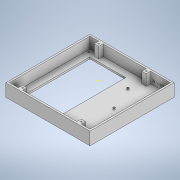
# Autodesk Inventor part: Backbox
Saved by Autodesk Inventor 2021 (Build 250183000, 183)
## iProperties
Created: 2022-08-07
Part Number: Backbox
Material: Generic
Document SubType Name: Modeling
Designer: Solom
Density: 1 g/cm^3
Appearance: Default
Author: Solom
Autodesk Inventor part; units mm, degrees
ref_plane "YZ Plane" through (0, 0, 0) normal (1, 0, 0) x (0, 1, 0)
ref_plane "XZ Plane" through (0, 0, 0) normal (0, 1, 0) x (-1, 0, 0)
ref_plane "XY Plane" through (0, 0, 0) normal (0, 0, 1) x (1, 0, 0)
sketch "Sketch1" plane through (0, 0, 0) normal (0, 1, 0) x (-1, 0, 0)
  line L0 (101.9092, 109.3301) -> (-90.0908, 109.3301)
  line L1 (-90.0908, 109.3301) -> (-90.0908, -82.6699)
  line L2 (-90.0908, -82.6699) -> (101.9092, -82.6699)
  line L3 (101.9092, -82.6699) -> (101.9092, 109.3301)
  line L4 (81.9092, 89.3301) -> (-70.0908, 89.3301)
  line L5 (-70.0908, 89.3301) -> (-70.0908, -62.6699)
  line L6 (-70.0908, -62.6699) -> (81.9092, -62.6699)
  line L7 (81.9092, -62.6699) -> (81.9092, 89.3301)
  point P0 (0, 0)
  dimension "d0" = 192
  dimension "d1" = 192
  dimension "d2" = 152
  dimension "d3" = 152
  dimension "d4" = 20
  dimension "d5" = 20
  constraints: 16 end point, 4 parallel, 2 horizontal, 2 perpendicular
  measures "d0" distance of L2.end L1.end
  measures "d1" distance of L1.end L0.end
  measures "d2" distance of L6.end L5.end
  measures "d3" distance of L5.end L4.end
  measures "d4" distance between parallel lines of L7 L3
  measures "d5" distance between parallel lines of L2 L6
extrude "Extrusion1" add sketch "Sketch1" along normal blind 4
sketch "Sketch2" plane through (0, 4, 0) normal (0, 1, 0) x (1, 0, 0)
  circle A0 centre (-92.4092, -96.8301) radius 1.5
  line L0 (-101.9092, -109.3301) -> (90.0908, -109.3301) projected
  line L1 (-101.9092, 82.6699) -> (-101.9092, -109.3301) projected
  circle A1 centre (-92.4092, 70.1699) radius 1.5
  line L2 (90.0908, 82.6699) -> (-101.9092, 82.6699) projected
  circle A2 centre (80.5908, 70.1699) radius 1.5
  line L3 (90.0908, -109.3301) -> (90.0908, 82.6699) projected
  circle A3 centre (80.5908, -96.8301) radius 1.5
  line L4 (-96.9092, 77.6699) -> (85.0908, 77.6699)
  line L5 (85.0908, 77.6699) -> (85.0908, -104.3301)
  line L6 (85.0908, -104.3301) -> (-96.9092, -104.3301)
  line L7 (-96.9092, -104.3301) -> (-96.9092, 77.6699)
  circle A4 centre (-84.4092, -101.8301) radius 1.25
  circle A5 centre (72.5908, 75.1699) radius 1.25
  point P0 (0, 0)
  dimension "d8" = 3
  dimension "d9" = 12.5
  dimension "d10" = 9.5
  dimension "d11" = 3
  dimension "d12" = 9.5
  dimension "d13" = 12.5
  dimension "d14" = 3
  dimension "d15" = 12.5
  dimension "d16" = 9.5
  dimension "d17" = 3
  dimension "d18" = 5
  dimension "d19" = 5
  dimension "d20" = 5
  dimension "d21" = 5
  dimension "d22" = 2.5
  dimension "d25" = 17.5
  dimension "d26" = 7.5
  dimension "d27" = 2.5
  dimension "d28" = 17.5
  dimension "d29" = 7.5
  constraints: 8 end point, 6 centre point, 2 parallel, 1 horizontal, 1 perpendicular
  measures "d8" diameter of A0
  measures "d9" distance from line of L0 A0.centre
  measures "d10" distance from line of L1 A0.centre
  measures "d11" diameter of A1
  measures "d12" distance from line of A1.centre L1
  measures "d13" distance from line of L2 A1.centre
  measures "d14" diameter of A2
  measures "d15" distance from line of L2 A2.centre
  measures "d16" distance from line of L3 A2.centre
  measures "d17" diameter of A3
  measures "d18" distance between parallel lines of L0 L6
  measures "d19" distance between parallel lines of L3 L5
  measures "d20" distance between parallel lines of L1 L7
  measures "d21" distance between parallel lines of L2 L4
  measures "d22" diameter of A4
  measures "d25" distance from line of L1 A4.centre
  measures "d26" distance from line of L0 A4.centre
  measures "d27" diameter of A5
  measures "d28" distance from line of L3 A5.centre
  measures "d29" distance from line of L2 A5.centre
hole "Hole1" at (80.5908, 4, 96.8301) at (-92.4092, 4, 96.8301) at (-92.4092, 4, -70.1699) at (80.5908, 4, -70.1699) direction (0, -1, 0) diameter 3 end through all
sketch "Sketch3" plane through (0, 4, 0) normal (0, 1, 0) x (1, 0, 0)
  circle A0 centre (-84.4092, -101.8301) radius 1.25
  line L0 (-101.9092, -109.3301) -> (90.0908, -109.3301) projected
  line L1 (-101.9092, 82.6699) -> (-101.9092, -109.3301) projected
  circle A1 centre (72.5908, 75.1699) radius 1.25
  line L2 (90.0908, 82.6699) -> (-101.9092, 82.6699) projected
  line L3 (90.0908, -109.3301) -> (90.0908, 82.6699) projected
  point P0 (0, 0)
  dimension "d37" = 2.5
  dimension "d38" = 7.5
  dimension "d39" = 17.5
  dimension "d40" = 2.5
  dimension "d41" = 7.5
  dimension "d42" = 17.5
  constraints: 2 centre point
  measures "d37" diameter of A0
  measures "d38" distance from line of L0 A0.centre
  measures "d39" distance from line of L1 A0.centre
  measures "d40" diameter of A1
  measures "d41" distance from line of L2 A1.centre
  measures "d42" distance from line of L3 A1.centre
hole "Hole2" at (-84.4092, 4, 101.8301) at (72.5908, 4, -75.1699) direction (0, -1, 0) diameter 2.5 end through all
sketch "Sketch4" plane through (0, 4, 0) normal (0, 1, 0) x (1, 0, 0)
  line L0 (-81.9092, 62.6699) -> (70.0908, 62.6699) projected
  line L1 (70.0908, 62.6699) -> (70.0908, -89.3301) projected
  line L2 (0, 62.6699) -> (70.0908, 62.6699)
  line L3 (70.0908, 62.6699) -> (70.0908, -89.3301)
  line L4 (70.0908, -89.3301) -> (0, -89.3301)
  line L5 (0, -89.3301) -> (0, 62.6699)
  point P0 (0, 0)
  constraints: 8 end point, 2 parallel, 1 horizontal, 1 perpendicular, 1 point on line
extrude "Extrusion2" add sketch "Sketch4" against normal blind 4
sketch "Sketch5" plane through (0, 4, 0) normal (0, 1, 0) x (1, 0, 0)
  circle A0 centre (25.7483, 41.7122) radius 1.5
  line L0 (25.7483, 41.7122) -> (49.2483, 41.7122)
  line L1 (49.2483, 41.7122) -> (49.2483, -13.3878)
  line L2 (49.2483, -13.3878) -> (25.7483, -13.3878)
  line L3 (25.7483, -13.3878) -> (25.7483, 41.7122)
  circle A1 centre (49.2483, -13.3878) radius 1.5
  point P0 (0, 0)
  dimension "d52" = 3
  dimension "d55" = 23.5
  dimension "d56" = 55.1
  dimension "d57" = 3
  constraints: 8 end point, 2 centre point, 2 parallel, 1 coincident, 1 horizontal, 1 perpendicular
  measures "d52" diameter of A0
  measures "d55" distance of L1.end L2.end
  measures "d56" distance of L0.end L1.end
  measures "d57" diameter of A1
hole "Hole3" at (25.7483, 4, -41.7122) at (49.2483, 4, 13.3878) direction (0, -1, 0) diameter 3 end through all
sketch "Sketch6" plane through (0, 4, 0) normal (0, 1, 0) x (1, 0, 0)
  line L0 (86.0908, 78.6699) -> (-97.9092, 78.6699)
  line L1 (-97.9092, 78.6699) -> (-97.9092, -105.3301)
  line L2 (-97.9092, -105.3301) -> (86.0908, -105.3301)
  line L3 (86.0908, -105.3301) -> (86.0908, 78.6699)
  line L4 (-101.9092, 82.6699) -> (-101.9092, -109.3301) projected
  line L5 (90.0908, 82.6699) -> (-101.9092, 82.6699) projected
  line L6 (90.0908, -109.3301) -> (90.0908, 82.6699) projected
  line L7 (-101.9092, -109.3301) -> (90.0908, -109.3301) projected
  line L8 (90.0908, 82.6699) -> (-101.9092, 82.6699) projected
  line L9 (90.0908, -109.3301) -> (90.0908, 82.6699) projected
  line L10 (-101.9092, 82.6699) -> (90.0908, 82.6699)
  line L11 (90.0908, 82.6699) -> (90.0908, -109.3301)
  line L12 (90.0908, -109.3301) -> (-101.9092, -109.3301)
  line L13 (-101.9092, -109.3301) -> (-101.9092, 82.6699)
  point P0 (0, 0)
  dimension "d65" = 4
  dimension "d66" = 4
  dimension "d67" = 4
  dimension "d68" = 4
  constraints: 16 end point, 4 parallel, 2 horizontal, 2 perpendicular
  measures "d65" distance between parallel lines of L1 L4
  measures "d66" distance between parallel lines of L5 L0
  measures "d67" distance between parallel lines of L6 L3
  measures "d68" distance between parallel lines of L7 L2
extrude "Extrusion3" add sketch "Sketch6" along normal blind 25
sketch "Sketch7" plane through (0, 29, 0) normal (0, 1, 0) x (1, 0, 0)
  point P0 (0, 0)
sketch "Sketch8" plane through (90.0908, 0, -82.6699) normal (0, 0, -1) x (-1, 0, 0)
  line L0 (18.4562, 10.3568) -> (27.5062, 10.3568)
  line L1 (27.5062, 10.3568) -> (27.5062, 14.9068)
  line L2 (27.5062, 14.9068) -> (18.4562, 14.9068)
  line L3 (18.4562, 14.9068) -> (18.4562, 10.3568)
  line L4 (27.5062, 12.6318) -> (31.6312, 12.6318)
  circle A0 centre (31.6312, 12.6318) radius 1.75
  line L5 (18.4562, 12.6318) -> (14.3312, 12.6318)
  circle A1 centre (14.3312, 12.6318) radius 1.75
  point P0 (90.0908, 0)
  dimension "d71" = 9.05
  dimension "d72" = 4.55
  dimension "d73" = 4.125
  dimension "d74" = 3.5
  dimension "d75" = 4.125
  dimension "d76" = 3.5
  constraints: 12 end point, 3 horizontal, 2 centre point, 2 coincident, 2 midpoint, 2 parallel, 1 perpendicular
  measures "d71" distance of L2.end L1.end
  measures "d72" distance of L1.end L0.end
  measures "d73" distance of L4.start L4.end
  measures "d74" diameter of A0
  measures "d75" distance of L5.start L5.end
  measures "d76" diameter of A1
extrude "Extrusion4" cut sketch "Sketch8" against normal blind 4
sketch "Sketch9" plane through (0, 29, 0) normal (0, 1, 0) x (1, 0, 0)
  point P0 (0, 0)
sketch "Sketch10" plane through (90.0908, 0, -82.6699) normal (0, 0, -1) x (-1, 0, 0)
  line L0 (27.5062, 10.3568) -> (27.5062, 14.9068) projected
  line L1 (27.5062, 12.6318) -> (42.7751, 12.6318)
  circle A0 centre (42.7751, 12.6318) radius 3.9
  point P0 (90.0908, 0)
  dimension "d79" = 7.8
  constraints: 2 end point, 1 centre point, 1 coincident, 1 horizontal, 1 midpoint
  measures "d79" diameter of A0
extrude "Extrusion5" cut sketch "Sketch10" against normal blind 1.5
sketch "Sketch11" plane through (47.3157, 12.6318, -81.1699) normal (0, 0, -1) x (-1, 0, 0)
  circle A0 centre (0, 0) radius 3.25
  point P0 (47.3157, -12.6318)
  dimension "d82" = 6.5
  constraints: 1 centre point
  measures "d82" diameter of A0
extrude "Extrusion6" cut sketch "Sketch11" against normal blind 2.5
sketch "Sketch12" plane through (0, 4, 0) normal (0, 1, 0) x (1, 0, 0)
  line L0 (-97.9092, 78.6699) -> (86.0908, 78.6699) projected
  line L1 (56.0908, 78.6699) -> (66.0908, 78.6699)
  line L2 (66.0908, 78.6699) -> (66.0908, 68.6699)
  line L3 (66.0908, 68.6699) -> (56.0908, 68.6699)
  line L4 (56.0908, 68.6699) -> (56.0908, 78.6699)
  line L5 (86.0908, 78.6699) -> (86.0908, -105.3301) projected
  line L6 (-97.9092, -105.3301) -> (86.0908, -105.3301) projected
  line L7 (66.0908, -105.3301) -> (56.0908, -105.3301)
  line L8 (56.0908, -105.3301) -> (56.0908, -95.3301)
  line L9 (56.0908, -95.3301) -> (66.0908, -95.3301)
  line L10 (66.0908, -95.3301) -> (66.0908, -105.3301)
  line L11 (-67.9092, 78.6699) -> (-77.9092, 78.6699)
  line L12 (-77.9092, 78.6699) -> (-77.9092, 68.6699)
  line L13 (-77.9092, 68.6699) -> (-67.9092, 68.6699)
  line L14 (-67.9092, 68.6699) -> (-67.9092, 78.6699)
  line L15 (-97.9092, -105.3301) -> (-97.9092, 78.6699) projected
  line L16 (-67.9092, -105.3301) -> (-77.9092, -105.3301)
  line L17 (-77.9092, -105.3301) -> (-77.9092, -95.3301)
  line L18 (-77.9092, -95.3301) -> (-67.9092, -95.3301)
  line L19 (-67.9092, -95.3301) -> (-67.9092, -105.3301)
  point P0 (0, 0)
  dimension "d85" = 10
  dimension "d86" = 10
  dimension "d87" = 20
  dimension "d88" = 10
  dimension "d89" = 10
  dimension "d90" = 10
  dimension "d91" = 10
  dimension "d92" = 20
  dimension "d93" = 10
  dimension "d94" = 10
  constraints: 32 end point, 8 parallel, 4 horizontal, 4 perpendicular, 4 point on line
  measures "d85" distance of L2.end L3.end
  measures "d86" distance of L1.end L2.end
  measures "d87" distance between parallel lines of L2 L5
  measures "d88" distance of L8.end L9.end
  measures "d89" distance of L7.end L8.end
  measures "d90" distance of L13.end L12.end
  measures "d91" distance of L12.end L11.end
  measures "d92" distance between parallel lines of L12 L15
  measures "d93" distance of L17.end L18.end
  measures "d94" distance of L16.end L17.end
extrude "Extrusion7" add sketch "Sketch12" along normal blind 25 contours L0 L14 L13 L12 | L17 L18 L19 L6 | L0 L2 L3 L4 | L8 L9 L10 L6
sketch "Sketch13" plane through (0, 29, 0) normal (0, 1, 0) x (1, 0, 0)
  line L0 (-67.9092, -95.3301) -> (-77.9092, -95.3301) projected
  line L1 (-72.9092, -95.3301) -> (-72.9092, -100.3301)
  circle A0 centre (-72.9092, -100.3301) radius 1.5
  line L2 (-67.9092, 68.6699) -> (-77.9092, 68.6699) projected
  line L3 (-72.9092, 68.6699) -> (-72.9092, 73.6699)
  line L4 (66.0908, 68.6699) -> (56.0908, 68.6699) projected
  line L5 (61.0908, 68.6699) -> (61.0908, 73.6699)
  line L6 (61.0908, -95.3301) -> (61.0908, -100.3301)
  circle A1 centre (61.0908, -100.3301) radius 1.5
  circle A2 centre (-72.9092, 73.6699) radius 1.5
  circle A3 centre (61.0908, 73.6699) radius 1.5
  point P0 (0, 0)
  dimension "d97" = 5
  dimension "d98" = 3
  dimension "d99" = 5
  dimension "d100" = 5
  dimension "d101" = 5
  dimension "d102" = 3
  dimension "d103" = 3
  dimension "d104" = 3
  constraints: 8 end point, 4 centre point, 4 coincident, 4 vertical, 3 midpoint
  measures "d97" distance of L1.start L1.end
  measures "d98" diameter of A0
  measures "d99" distance of L3.start L3.end
  measures "d100" distance of L5.start L5.end
  measures "d101" distance of L6.start L6.end
  measures "d102" diameter of A1
  measures "d103" diameter of A2
  measures "d104" diameter of A3
hole "Hole4" at (-72.9092, 29, -73.6699) at (-72.9092, 29, 100.3301) at (61.0908, 29, 100.3301) at (61.0908, 29, -73.6699) direction (0, -1, 0) diameter 3 depth 6 tip angle 118
sketch "Sketch14" plane through (-67.9092, 4, -78.6699) normal (0, 0, 1) x (1, 0, 0)
  point P0 (67.9092, -4)
sketch "Sketch15" plane through (0, 29, 0) normal (0, 1, 0) x (1, 0, 0)
  line L0 (56.0908, 78.6699) -> (56.0908, 68.6699) projected
  line L1 (66.0908, 68.6699) -> (66.0908, 78.6699) projected
  line L2 (56.0908, 78.6699) -> (66.0908, 78.6699)
  line L3 (66.0908, 78.6699) -> (71.6345, 78.6699) projected
  line L4 (56.0908, 68.6699) -> (66.0908, 68.6699)
  line L5 (66.0908, 68.6699) -> (66.0908, 78.6699)
  line L6 (66.0908, 78.6699) -> (56.0908, 78.6699)
  line L7 (56.0908, 78.6699) -> (56.0908, 68.6699)
  point P0 (0, 0)
  constraints: 10 end point, 2 parallel, 2 perpendicular, 1 horizontal
extrude "Extrusion8" cut sketch "Sketch15" against normal blind 25
sketch "Sketch16" plane through (0, 4, 0) normal (0, 1, 0) x (1, 0, 0)
  line L0 (86.0908, 78.6699) -> (-67.9092, 78.6699) projected
  line L1 (30.7253, 78.6699) -> (40.7253, 78.6699)
  line L2 (40.7253, 78.6699) -> (40.7253, 68.6699)
  line L3 (40.7253, 68.6699) -> (30.7253, 68.6699)
  line L4 (30.7253, 68.6699) -> (30.7253, 78.6699)
  point P0 (0, 0)
  dimension "d114" = 10
  dimension "d115" = 10
  constraints: 8 end point, 2 parallel, 1 horizontal, 1 perpendicular, 1 point on line
  measures "d114" distance of L2.end L3.end
  measures "d115" distance of L1.end L2.end
extrude "Extrusion9" add sketch "Sketch16" along normal blind 25
sketch "Sketch17" plane through (0, 29, 0) normal (0, 1, 0) x (1, 0, 0)
  line L0 (30.7253, 68.6699) -> (40.7253, 68.6699) projected
  line L1 (35.7253, 68.6699) -> (35.7253, 73.6699)
  circle A0 centre (35.7253, 73.6699) radius 1.5
  point P0 (0, 0)
  dimension "d118" = 5
  dimension "d119" = 3
  constraints: 2 end point, 1 centre point, 1 coincident, 1 midpoint, 1 vertical
  measures "d118" distance of L1.start L1.end
  measures "d119" diameter of A0
hole "Hole5" at (35.7253, 29, -73.6699) direction (0, -1, 0) diameter 3 depth 6 tip angle 118
sketch "Sketch18" plane through (0, 4, 0) normal (0, 1, 0) x (1, 0, 0)
  circle A0 centre (25.7483, 41.7122) radius 1.5 projected
  circle A1 centre (25.7483, 41.7122) radius 2.5
  circle A2 centre (49.2483, -13.3878) radius 1.5 projected
  circle A3 centre (49.2483, -13.3878) radius 2.5
  point P0 (0, 0)
  dimension "d127" = 5
  dimension "d128" = 5
  constraints: 2 centre point, 2 coincident
  measures "d127" diameter of A1
  measures "d128" diameter of A3
extrude "Extrusion10" add sketch "Sketch18" along normal blind 3 contours A1
sketch "Sketch19" plane through (0, 4, 0) normal (0, 1, 0) x (1, 0, 0)
  circle A0 centre (49.2483, -13.3878) radius 1.5 projected
  circle A1 centre (49.2483, -13.3878) radius 2.5
  point P0 (0, 0)
  dimension "d131" = 5
  constraints: 1 centre point, 1 coincident
  measures "d131" diameter of A1
extrude "Extrusion11" add sketch "Sketch19" along normal blind 3
body "Solid1"
